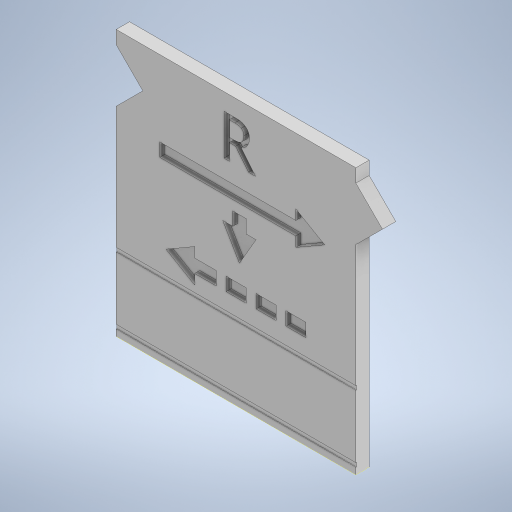
# Autodesk Inventor part: MS_R[203] text 80x60
Saved by Autodesk Inventor 2024 (Build 280153000, 153)
## iProperties
Created: 2023-03-29
Part Number: MS_R[203] text 80x60
Material: Generic
Document SubType Name: Modeling
Designer: LKLM8608
Density: 1 g/cm^3
Appearance: Default
Author: LKLM8608
Autodesk Inventor part; units mm, degrees
ref_plane "YZ Plane" through (0, 0, 0) normal (1, 0, 0) x (0, 1, 0)
ref_plane "XZ Plane" through (0, 0, 0) normal (0, 1, 0) x (-1, 0, 0)
sketch "Sketch1" plane through (0, 0, 0) normal (0, 0, 1) x (1, 0, 0)
  line L0 (6.0134, 0.5413) -> (-66.0587, 0.5413)
  circle A0 centre (-66.0587, 68.5413) radius 8 construction
  line L1 (-66.0587, 60.5413) -> (6.0134, 60.5413) construction
  line L2 (-66.0587, 76.5413) -> (-58.0587, 68.5413)
  line L3 (-66.0587, 60.5413) -> (-58.0587, 68.5413)
  line L4 (6.0134, 60.5413) -> (6.0134, 0.5413)
  line L5 (-66.0587, 0.5413) -> (-66.0587, 60.5413)
  line L6 (-66.0587, 76.5413) -> (-66.0587, 80.5413)
  line L7 (6.0134, 0.5413) -> (-120, 0.5413) construction
  line L8 (-60, 0) -> (-60, 75) construction
  line L9 (-60, 75) -> (0, 75) construction
  line L10 (6.0134, 150.5413) -> (6.0134, 0.5413) construction
  line L11 (6.0134, 60.5413) -> (6.0134, 80.5413)
  line L12 (-66.0587, 80.5413) -> (6.0134, 80.5413)
  line L13 (-66.0587, 76.5413) -> (12.8048, 76.5413) construction
  line L14 (-58.0587, 68.5413) -> (17.3629, 68.5413) construction
  line L15 (-66.0587, 60.5413) -> (24.3855, 60.5413) construction
  circle A1 centre (6.0134, 68.5413) radius 8 construction
  line L16 (6.0134, 60.5413) -> (14.0134, 68.5413)
  line L17 (14.0134, 68.5413) -> (6.0134, 76.5413)
  point P0 (0, 0)
  dimension "d1" = 80
  dimension "d5" = 16
  dimension "d6" = 60
  constraints: 36 end point, 6 point on line, 5 horizontal, 5 point on circle, 4 parallel, 4 perpendicular, 3 tangent, 2 centre point
  measures "d1" distance of L0.end L6.end
  measures "d5" diameter of A0
  measures "d6" distance between parallel lines of L0 L1
extrude "Extrusion1" add sketch "Sketch1" along normal blind 4
sketch "Sketch3" plane through (0, 0, 4) normal (0, 0, 1) x (1, 0, 0)
  line L0 (-66.0587, 80.5413) -> (13.9413, 80.5413) construction
  line L1 (-34.8487, 75.4475) -> (-28.5043, 75.4475) construction
  line L2 (-28.5043, 75.4475) -> (-28.5043, 84.7097) construction
  line L3 (-28.5043, 84.7097) -> (-34.8487, 84.7097) construction
  line L4 (-34.8487, 84.7097) -> (-34.8487, 75.4475) construction
  line L5 (-52.9694, 57.7889) -> (-12.0353, 57.7889)
  line L6 (-12.0353, 57.7889) -> (-12.0353, 60.7889)
  line L7 (-12.0353, 60.7889) -> (-3.3751, 55.7889)
  line L8 (-12.0353, 50.7889) -> (-3.3751, 55.7889)
  line L9 (-12.0353, 50.7889) -> (-12.0353, 53.7889)
  line L10 (-52.9694, 53.7889) -> (-12.0353, 53.7889)
  line L11 (-52.9694, 57.7889) -> (-52.9694, 53.7889)
  line L12 (-27, 50.7889) -> (-31, 50.7889)
  line L13 (-31, 50.7889) -> (-31, 46.7889)
  line L14 (-27, 46.7889) -> (-27, 50.7889)
  line L15 (-27, 50.7889) -> (-27, 52.7889) construction
  line L16 (-27, 35.7889) -> (-27, 32.7889) construction
  line L17 (-27, 32.7889) -> (-33, 32.7889)
  line L18 (-33, 32.7889) -> (-33, 28.7889)
  line L19 (-33, 28.7889) -> (-27, 28.7889)
  line L20 (-27, 28.7889) -> (-27, 32.7889)
  line L21 (-33, 32.7889) -> (-36, 32.7889) construction
  line L22 (-36, 32.7889) -> (-36, 28.7889)
  line L23 (-36, 32.7889) -> (-42.4587, 32.7889)
  line L24 (-42.4587, 32.7889) -> (-42.4587, 35.7889)
  line L25 (-42.4587, 35.7889) -> (-51.0587, 30.7889)
  line L26 (-36, 28.7889) -> (-42.4587, 28.7889)
  line L27 (-42.4587, 28.7889) -> (-42.4587, 25.7889)
  line L28 (-42.4587, 25.7889) -> (-51.0587, 30.7889)
  line L29 (6.0134, 0.5413) -> (-66.0587, 0.5413) construction
  line L30 (-66.0587, 80.5413) -> (6.0134, 80.5413) construction
  line L31 (-30.0226, 80.5413) -> (-30.0226, 0.5413) construction
  line L32 (-24, 32.7889) -> (-18, 32.7889)
  line L33 (-18, 32.7889) -> (-18, 28.7889)
  line L34 (-18, 28.7889) -> (-24, 28.7889)
  line L35 (-24, 28.7889) -> (-24, 32.7889)
  line L36 (-15, 32.7889) -> (-9, 32.7889)
  line L37 (-9, 32.7889) -> (-9, 28.7889)
  line L38 (-9, 28.7889) -> (-15, 28.7889)
  line L39 (-15, 28.7889) -> (-15, 32.7889)
  line L40 (-27, 46.7889) -> (-24, 46.7889)
  line L41 (-31, 46.7889) -> (-34, 46.7889)
  line L42 (-66.0587, 0.5413) -> (-66.0587, 60.5413) construction
  line L43 (6.0134, 60.5413) -> (6.0134, 0.5413) construction
  line L44 (-29, 50.7889) -> (-29, 38.1889) construction
  line L45 (-34, 46.7889) -> (-29, 38.1889)
  line L46 (-24, 46.7889) -> (-29, 38.1889)
  line L47 (-24.1712, 63.2475) -> (-26.277, 63.2475)
  line L48 (-26.277, 63.2475) -> (-30.1328, 68.1018)
  line L49 (-30.1328, 68.1018) -> (-31.9915, 68.1018)
  line L50 (-31.9915, 68.1018) -> (-31.9915, 63.2475)
  line L51 (-31.9915, 63.2475) -> (-33.6129, 63.2475)
  line L52 (-33.6129, 63.2475) -> (-33.6129, 75.4475)
  line L53 (-33.6129, 75.4475) -> (-30.4689, 75.4475)
  spline S0 degree 2 poles (-30.4689, 75.4475) (-29.421, 75.4475) (-28.0072, 75.2201) (-27.3646, 74.8048) knots 0 0 0 1 2 2 2
  spline S1 degree 2 poles (-27.3646, 74.8048) (-26.7219, 74.3896) (-25.9804, 73.0945) (-25.9804, 72.1355) knots 0 0 0 1 2 2 2
  spline S2 degree 2 poles (-25.9804, 72.1355) (-25.9804, 70.8008) (-27.3448, 68.9915) (-28.5114, 68.5565) knots 0 0 0 1 2 2 2
  line L54 (-28.5114, 68.5565) -> (-24.1712, 63.2475)
  spline S3 degree 2 poles (-27.671, 72.0069) (-27.671, 72.5408) (-28.0467, 73.3614) (-28.4422, 73.6283) knots 0 0 0 1 2 2 2
  spline S4 degree 2 poles (-28.4422, 73.6283) (-28.7882, 73.8557) (-29.7077, 74.0436) (-30.38, 74.0436) knots 0 0 0 1 2 2 2
  line L55 (-30.38, 74.0436) -> (-31.9915, 74.0436)
  line L56 (-31.9915, 74.0436) -> (-31.9915, 69.4562)
  line L57 (-31.9915, 69.4562) -> (-30.5678, 69.4562)
  spline S5 degree 2 poles (-30.5678, 69.4562) (-29.8659, 69.4562) (-28.7487, 69.7034) (-28.3631, 70.089) knots 0 0 0 1 2 2 2
  spline S6 degree 2 poles (-28.3631, 70.089) (-28.0072, 70.4251) (-27.671, 71.3742) (-27.671, 72.0069) knots 0 0 0 1 2 2 2
  point P0 (-26.0587, 80.5413)
  point P1 (-12.0353, 60.7889)
  point P2 (-42.4587, 34.2889)
  point P3 (6.0134, 30.5413)
  point P4 (-9, 30.7889)
  point P5 (-25.5, 46.7889)
  dimension "d65" = 4
  dimension "d66" = 3
  dimension "d67" = 10
  dimension "d68" = 3
  dimension "d88" = 4
  dimension "d92" = 6
  dimension "d93" = 4
  dimension "d94" = 3
  dimension "d96" = 3
  dimension "d97" = 3
  dimension "d121" = 6
  dimension "d122" = 4
  dimension "d123" = 6
  dimension "d124" = 3
  dimension "d125" = 3
  dimension "d128" = 3
  dimension "d130" = 4
  dimension "d132" = 3
  dimension "d133" = 3
  dimension "d134" = 8.6
  dimension "d135" = 15
  dimension "d136" = 15.0134
  dimension "d137" = 12.6
  dimension "d138" = 4
  constraints: 76 end point, 8 horizontal, 8 midpoint, 8 parallel, 6 vertical, 5 perpendicular, 2 point on line, 2 other
  measures "d65" distance of L5.end L9.end
  measures "d66" distance of L5.end L6.end
  measures "d67" distance of L6.end L7.end
  measures "d68" distance of L9.end L8.start
  measures "d88" distance of L13.end L12.end
  measures "d92" distance of L19.end L18.end
  measures "d93" distance of L18.end L17.end
  measures "d94" distance of L17.end L21.end
  measures "d96" distance of L23.end L24.end
  measures "d97" distance of L26.end L27.end
  measures "d121" distance of L33.end L34.end
  measures "d122" distance of L32.end L33.end
  measures "d123" distance of L37.end L38.end
  measures "d124" distance between parallel lines of L20 L35
  measures "d125" distance between parallel lines of L33 L39
  measures "d128" distance between parallel lines of L12 L10
  measures "d130" distance between parallel lines of L13 L14
  measures "d132" distance of L14.start L40.end
  measures "d133" distance of L13.end L41.end
  measures "d134" horizontal distance of L25.end point (-42.459, 34.289)
  measures "d135" distance from line of L42 L25.end
  measures "d136" horizontal distance of point (6.013, 30.541) point (-9, 30.789)
  measures "d137" distance of L44.start L44.end
  measures "d138" vertical distance of L12.start point (-25.5, 46.789)
extrude "Extrusion3" cut sketch "Sketch3" against normal blind 1.5
ref_plane "Work Plane2" through (0, 0, 0.4) normal (0, 0, -1) x (-1, 0, 0)
sketch "Sketch5" plane through (0, 0, 0.4) normal (0, 0, -1) x (-1, 0, 0)
  line L0 (-13.9413, 80.5413) -> (66.0587, 80.5413) construction
  line L1 (-6.0134, 0.5413) -> (-6.0134, 76.5413) construction
  line L2 (66.0587, 0.5413) -> (-6.0134, 0.5413) construction
  line L3 (66.0587, 60.5413) -> (66.0587, 0.5413) construction
  line L4 (66.0587, 80.5413) -> (66.0587, 76.5413) construction
  line L5 (-6.0134, 0.5413) -> (-6.0134, 60.5413) construction
  line L6 (66.0587, 0.5413) -> (-6.0134, 0.5413) construction
  line L7 (66.0587, 60.5413) -> (66.0587, 0.5413) construction
  line L8 (58.0587, 68.5413) -> (66.0587, 60.5413) construction
  line L9 (66.0587, 76.5413) -> (58.0587, 68.5413) construction
  circle A0 centre (30.0226, 14.5413) radius 3.075
  line L10 (31, 46.7889) -> (31, 50.7889) construction
  line L11 (31, 50.7889) -> (27, 50.7889) construction
  line L12 (27, 50.7889) -> (27, 46.7889) construction
  line L13 (3.3751, 55.7889) -> (12.0353, 50.7889) construction
  line L14 (12.0353, 50.7889) -> (12.0353, 53.7889) construction
  line L15 (12.0353, 53.7889) -> (52.9694, 53.7889) construction
  line L16 (52.9694, 53.7889) -> (52.9694, 57.7889) construction
  line L17 (52.9694, 57.7889) -> (12.0353, 57.7889) construction
  line L18 (12.0353, 57.7889) -> (12.0353, 60.7889) construction
  line L19 (12.0353, 60.7889) -> (3.3751, 55.7889) construction
  line L20 (42.4587, 25.7889) -> (51.0587, 30.7889) construction
  line L21 (51.0587, 30.7889) -> (42.4587, 35.7889) construction
  line L22 (42.4587, 35.7889) -> (42.4587, 32.7889) construction
  line L23 (42.4587, 32.7889) -> (36, 32.7889) construction
  line L24 (36, 32.7889) -> (36, 28.7889) construction
  line L25 (36, 28.7889) -> (42.4587, 28.7889) construction
  line L26 (42.4587, 28.7889) -> (42.4587, 25.7889) construction
  line L27 (27, 28.7889) -> (33, 28.7889) construction
  line L28 (33, 28.7889) -> (33, 32.7889) construction
  line L29 (33, 32.7889) -> (27, 32.7889) construction
  line L30 (27, 32.7889) -> (27, 28.7889) construction
  line L31 (66.0587, 76.5413) -> (66.0587, 80.5413) construction
  line L32 (58.0587, 68.5413) -> (66.0587, 76.5413) construction
  line L33 (66.0587, 60.5413) -> (58.0587, 68.5413) construction
  line L34 (66.0587, 0.5413) -> (66.0587, 60.5413) construction
  line L35 (-6.0134, 0.5413) -> (66.0587, 0.5413) construction
  line L36 (-6.0134, 60.5413) -> (-6.0134, 0.5413) construction
  line L37 (-6.0134, 80.5413) -> (66.0587, 80.5413) projected
  line L38 (66.0587, 80.5413) -> (-6.0134, 80.5413) projected
  line L39 (-6.0134, 76.5413) -> (-6.0134, 80.5413) projected
  line L40 (-14.0134, 68.5413) -> (-6.0134, 76.5413) projected
  line L41 (-6.0134, 60.5413) -> (-14.0134, 68.5413) projected
  line L42 (-14.0134, 68.5413) -> (-6.0134, 60.5413) projected
  line L43 (-6.0134, 76.5413) -> (-14.0134, 68.5413) projected
  line L44 (-6.0134, 80.5413) -> (-6.0134, 76.5413) projected
  line L45 (27, 46.7889) -> (24, 46.7889) projected
  line L46 (24, 46.7889) -> (29, 38.1889) projected
  line L47 (29, 38.1889) -> (34, 46.7889) projected
  line L48 (34, 46.7889) -> (31, 46.7889) projected
  dimension "d99" = 80
  dimension "d100" = 72.0721
  dimension "d101" = 6.15
  dimension "d102" = 14
  dimension "d103" = 36.036
  constraints: 1 centre point, 1 other
  measures "d99" distance between parallel lines of L0 L2
  measures "d101" diameter of A0
  measures "d102" distance from line of L2 A0.centre
  measures "d103" distance from line of L3 A0.centre
extrude "Extrusion4" cut sketch "Sketch5" against normal blind 3.15
sketch "Sketch7" plane through (0, 0, 4) normal (0, 0, 1) x (1, 0, 0)
  line L0 (-66.0587, 0.5413) -> (-66.0587, 60.5413) construction
  line L1 (6.0134, 0.5413) -> (-66.0587, 0.5413) construction
  line L2 (6.0134, 80.5413) -> (6.0134, 0.5413) construction
  line L3 (-58.2371, 23.7889) -> (9.8349, 23.7889)
  line L4 (6.0134, 2.5413) -> (-64.0587, 2.5413)
  line L5 (7.8349, 22.5889) -> (-56.2371, 22.5889)
  line L6 (-62.0587, 3.7413) -> (2.0134, 3.7413)
  line L7 (-56.2371, 22.5889) -> (-58.2371, 22.5889)
  line L8 (7.8349, 22.5889) -> (9.8349, 22.5889)
  line L9 (2.0134, 3.7413) -> (4.0134, 3.7413)
  line L10 (-62.0587, 3.7413) -> (-64.0587, 3.7413)
  line L11 (-58.2371, 23.7889) -> (-66.0587, 23.7889)
  line L12 (-58.2371, 22.5889) -> (-66.0587, 22.5889)
  line L13 (-66.0587, 23.7889) -> (-66.0587, 22.5889)
  line L14 (-64.0587, 3.7413) -> (-66.0587, 3.7413)
  line L15 (-64.0587, 2.5413) -> (-66.0587, 2.5413)
  line L16 (-66.0587, 3.7413) -> (-66.0587, 2.5413)
  line L17 (9.8349, 23.7889) -> (6.0134, 23.7889)
  line L18 (9.8349, 22.5889) -> (6.0134, 22.5889)
  line L19 (6.0134, 23.7889) -> (6.0134, 22.5889)
  line L20 (4.0134, 3.7413) -> (6.0134, 3.7413)
  line L21 (6.0134, 3.7413) -> (6.0134, 2.5413)
  point P0 (-42.4587, 25.7889)
  point P1 (6.0134, 60.5413)
  point P2 (0, 0)
  dimension "d115" = 2
  dimension "d116" = 2
  dimension "d117" = 1.2
  dimension "d120" = 1.2
  constraints: 38 end point, 10 point on line, 5 perpendicular, 4 parallel, 2 collinear, 2 horizontal, 2 vertical
  measures "d115" distance between parallel lines of L1 L4
  measures "d116" distance from line of point (-42.459, 25.789) L3
  measures "d117" distance between parallel lines of L3 L5
  measures "d120" distance between parallel lines of L4 L6
extrude "Extrusion5" cut sketch "Sketch7" against normal blind 0.2
sketch "Sketch8" plane through (-66.0587, 0.5413, 0) normal (0, -1, 0) x (1, 0, 0)
  line L0 (72.0721, 4) -> (0, 4) construction
  line L1 (0, 0) -> (0, 4) construction
  line L2 (0, 0) -> (72.0721, 0) construction
  line L3 (72.0721, 0) -> (72.0721, 4) construction
  line L4 (72.0721, 4) -> (0, 4) construction
  line L5 (0, 0) -> (0, 4) construction
  line L6 (0, 0) -> (72.0721, 0) construction
  line L7 (72.0721, 0) -> (72.0721, 4) construction
  point P0 (66.0587, 0)
body "Solid1"
